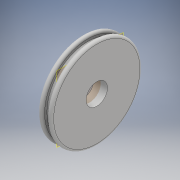
# Autodesk Inventor part: rueda servo
Saved by Autodesk Inventor 2018 (Build 220112000, 112)
## iProperties
Created: 2018-02-25
Part Number: rueda servo
Material: Genérico
Document SubType Name: Modeling
Designer: ivanb
Density: 1 g/cm^3
Appearance: Valor por defecto
Author: ivanb
Autodesk Inventor part; units mm, degrees
ref_plane "YZ Plane" through (0, 0, 0) normal (1, 0, 0) x (0, 1, 0)
ref_plane "XZ Plane" through (0, 0, 0) normal (0, 1, 0) x (-1, 0, 0)
ref_plane "XY Plane" through (0, 0, 0) normal (0, 0, 1) x (1, 0, 0)
sketch "Boceto1" plane through (0, 0, 0) normal (1, 0, 0) x (0, 1, 0)
  circle A0 centre (0, 0) radius 10
  dimension "d2" = 20
  constraints: 1 centre point, 1 coincident
  measures "d2" diameter of A0
extrude "Extrusión1" add sketch "Boceto1" along normal blind 3
ref_plane "Plano de trabajo1" through (1.5, 0, 0) normal (1, 0, 0) x (0, 0, -1)
sketch "Boceto2" plane through (1.5, 0, 0) normal (1, 0, 0) x (0, 0, -1)
  circle A0 centre (0, 0) radius 14.342
  circle A1 centre (0, 0) radius 9
  dimension "d3" = 18
  constraints: 2 centre point, 2 coincident
  measures "d3" diameter of A1
extrude "Extrusión2" cut sketch "Boceto2" along normal blind 0.5 and the other way blind 0.5
fillet "Empalme1" radius 0.5 4 edges at (3, -10, 0) (2, -10, 0) (1, -10, 0) (0, -10, 0)
sketch "Boceto3" plane through (3, 0, 0) normal (1, 0, 0) x (0, 0, -1)
  circle A0 centre (0, 0) radius 2.35
  dimension "d9" = 4.7
  constraints: 1 centre point, 1 coincident
  measures "d9" diameter of A0
extrude "Extrusión3" cut sketch "Boceto3" against normal blind 10
